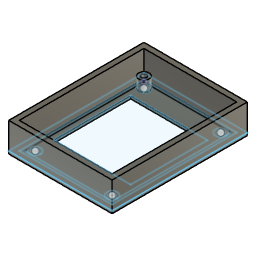
TFT Display Holder v1 (Autodesk Fusion 360 design; units mm, degrees)
Autodesk Fusion 360 part; units mm, degrees
sketch "Sketch1" plane through (0, 0, 0) normal (0, 0, 1) x (1, 0, 0)
  line L0 (0, 0) -> (33, 0)
  line L1 (33, 0) -> (33, -45)
  line L2 (33, -45) -> (0, -45)
  line L3 (0, -45) -> (0, 0)
  circle A0 centre (31, -2) radius 1
  circle A1 centre (2, -2) radius 1
  circle A2 centre (2, -43) radius 1
  circle A3 centre (31, -43) radius 1
  line L4 (34, 1) -> (34, -46)
  line L5 (34, -46) -> (-1, -46)
  line L6 (-1, -46) -> (-1, 1)
  line L7 (-1, 1) -> (34, 1)
  line L8 (36, 3) -> (36, -48)
  line L9 (36, -48) -> (-3, -48)
  line L10 (-3, -48) -> (-3, 3)
  line L11 (-3, 3) -> (36, 3)
  circle A4 centre (31, -2) radius 2
  circle A5 centre (31, -43) radius 2
  circle A6 centre (2, -43) radius 2
  circle A7 centre (2, -2) radius 2
  line L12 (31, -36) -> (2, -36)
  line L13 (2, -36) -> (2, -7)
  line L14 (2, -7) -> (31, -7)
  line L15 (31, -7) -> (31, -36)
  constraint horizontal L0
  constraint vertical L1
  constraint horizontal L2
  constraint vertical L3
  constraint coincident L0.start L3.end
  constraint parallel L1 L4
  constraint perpendicular L4 L5
  constraint perpendicular L5 L6
  constraint perpendicular L4 L7
  constraint perpendicular L7 L8
  constraint perpendicular L8 L9
  constraint perpendicular L9 L10
  constraint perpendicular L8 L11
  constraint concentric A0 A4
  constraint tangent L1 A4
  constraint concentric A3 A5
  constraint tangent L1 A5
  constraint concentric A2 A6
  constraint concentric A1 A7
  constraint perpendicular L4 L12
  constraint perpendicular L12 L13
  constraint perpendicular L13 L14
  constraint perpendicular L12 L15
extrude "Extrude1" add sketch "Sketch1" along normal blind 20 contours L8 L9 L10 L11 makes body 1
extrude "Extrude2" add sketch "Sketch1" along normal blind 4 separate body contours A7 | A4 | A6 | A5 makes body 2 at (32.9975, -43.0997, 1.3333) makes body 3 at (0.6766, -41.5004, 2.6667) makes body 4 at (32.9975, -2.0997, 1.3333) makes body 5 at (3.9975, -2.0997, 1.3333)
extrude "Extrude3" add sketch "Sketch1" against normal blind 1 contours L0 L3 A7 | L0 L1 L2 L3 A4 A5 A6 A7 | A7 | L0 L1 A4 | A4 | L2 L3 A6 | A6 | A5 | L1 L2 A5 | A0 | A1 | A2 | A3 | L4 L5 L6 L7 | L8 L9 L10 L11 bodies 1 2 3 4 5
extrude "Extrude4" cut 1 faces at (35.3333, -30.3333, 20) along direction (0, 0, -1) blind 10 on bodies 1 bodies 1
